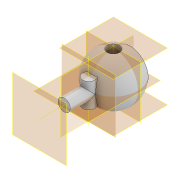
# Autodesk Inventor part: ChestP
Saved by Autodesk Inventor 2021 (Build 250183000, 183)
## iProperties
Created: 2020-12-19
Part Number: ChestP
Material: 一般
Document SubType Name: Modeling
Designer: Tazaki
Density: 1.30491 g/cm^3
Appearance: 既定
Mass: 5000 g
Surface Area: 1711.42 cm^2
Volume: 3831.68 cm^3
Author: Tazaki
Autodesk Inventor part; units mm, degrees
sketch "スケッチ1" plane through (0, 0, 0) normal (0, 0, 1) x (1, 0, 0)
  arc A0 (0, 100) -> (0, -100) centre (0, 0) ccw
  line L0 (0, 100) -> (0, -100)
  dimension "d0" = 200
  constraints: 2 end point, 2 point on circle, 1 centre point, 1 coincident, 1 vertical
  measures "d0" diameter of A0
revolve "回転1" add sketch "スケッチ1" angle 360 about axis through (0, 100, 0) along (0, -1, 0)
ref_plane "作業平面1" through (0, 0, 300) normal (0, 0, 1) x (1, 0, 0)
ref_plane "作業平面2" through (0, 100, 0) normal (0, 1, 0) x (-1, 0, 0)
ref_plane "作業平面3" through (0, -100, 0) normal (0, 1, 0) x (-1, 0, 0)
ref_plane "作業平面4" through (0, 0, 100) normal (0, 0, 1) x (1, 0, 0)
sketch "スケッチ2" plane through (0, 0, 0) normal (1, 0, 0) x (0, 1, 0)
  line L0 (134.8667, -67.7722) -> (-130.8003, -67.7722)
  line L1 (-130.8003, -67.7722) -> (-130.8003, -136.448)
  line L2 (-130.8003, -136.448) -> (134.8667, -136.448)
  line L3 (134.8667, -136.448) -> (134.8667, -67.7722)
  point P0 (0, 0)
  constraints: 8 end point, 2 parallel, 1 horizontal, 1 perpendicular
extrude "押し出し1" cut sketch "スケッチ2" along normal mid plane 200
sketch "スケッチ3" plane through (0, 0, 0) normal (0, 1, 0) x (-1, 0, 0)
  circle A0 centre (0, 0) radius 25
  dimension "d8" = 50
  constraints: 1 centre point, 1 coincident
  measures "d8" diameter of A0
extrude "押し出し2" cut sketch "スケッチ3" along normal mid plane 200
sketch "スケッチ4" plane through (0, 0, 0) normal (0, 0, 1) x (1, 0, 0)
  circle A0 centre (0, 0) radius 25
  dimension "d11" = 50
  constraints: 1 centre point, 1 coincident
  measures "d11" diameter of A0
extrude "押し出し3" add sketch "スケッチ4" along normal blind 200
sketch "スケッチ5" plane through (0, 0, 0) normal (0, 1, 0) x (-1, 0, 0)
  circle A0 centre (0, 100) radius 25
  point P0 (0, 0)
  dimension "d14" = 50
  dimension "d15" = 100
  constraints: 1 centre point, 1 vertical alignment
  measures "d14" diameter of A0
  measures "d15" distance of A0.centre point (0, 0)
extrude "押し出し4" add sketch "スケッチ5" along normal mid plane 100
